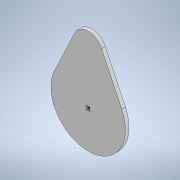
# Autodesk Inventor part: 4.2 Part D
Saved by Autodesk Inventor 2020 (Build 240168000, 168)
## iProperties
Created: 2020-01-07
Part Number: 4.2 Part D
Material: Generic
Document SubType Name: Modeling
Designer: cks4a449
Density: 1 g/cm^3
Appearance: Default
Author: cks4a449
Autodesk Inventor part; units mm, degrees
ref_plane "YZ Plane" through (0, 0, 0) normal (1, 0, 0) x (0, 1, 0)
ref_plane "XZ Plane" through (0, 0, 0) normal (0, 1, 0) x (-1, 0, 0)
ref_plane "XY Plane" through (0, 0, 0) normal (0, 0, 1) x (1, 0, 0)
sketch "Sketch1" plane through (0, 0, 0) normal (0, 0, 1) x (1, 0, 0)
  line L0 (0, 0) -> (0, 1.5875)
  line L1 (-1.5875, 1.5875) -> (1.5875, 1.5875)
  line L2 (1.5875, 1.5875) -> (1.5875, -1.5875)
  line L3 (1.5875, -1.5875) -> (-1.5875, -1.5875)
  line L4 (-1.5875, -1.5875) -> (-1.5875, 1.5875)
  line L5 (-1.5875, 1.5875) -> (1.5875, -1.5875) construction
  line L6 (1.5875, 1.5875) -> (-1.5875, -1.5875) construction
  arc A0 (11.4746, 49.8929) -> (-11.4746, 49.8929) centre (0, 44.45) ccw
  arc A1 (-28.6864, 13.6071) -> (28.6864, 13.6071) centre (0, 0) ccw
  line L7 (-11.4746, 49.8929) -> (-28.6864, 13.6071)
  line L8 (11.4746, 49.8929) -> (28.6864, 13.6071)
  dimension "d3" = 3.175
  dimension "d4" = 3.175
  dimension "d9" = 44.45
  constraints: 18 end point, 4 point on circle, 4 tangent, 3 midpoint, 2 centre point, 2 parallel, 1 coincident, 1 horizontal, 1 perpendicular, 1 vertical
  measures "d3" distance of L2.end L3.end
  measures "d4" distance of L1.end L2.end
  measures "d9" distance of L0.start A0.centre
extrude "Extrusion1" add sketch "Sketch1" along normal blind 3.175
body "Solid1"
